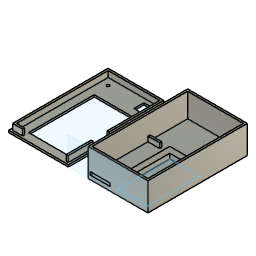
Untitled v1 (Autodesk Fusion 360 design; units mm, degrees)
Autodesk Fusion 360 part; units mm, degrees
sketch "Sketch1" plane through (0, 0, 0) normal (0, 0, 1) x (1, 0, 0)
  line L0 (0, 0) -> (76.2, 0)
  line L1 (76.2, 0) -> (76.2, 127)
  line L2 (76.2, 127) -> (0, 127)
  line L3 (0, 127) -> (0, 0)
  constraint horizontal L0
  constraint vertical L1
  constraint horizontal L2
  constraint vertical L3
  constraint coincident L0.start L3.end
extrude "Extrude1" add sketch "Sketch1" along normal blind 35.56 makes body 1
sketch "Sketch2" plane through (0, 0, 35.56) normal (0, 0, 1) x (-1, 0, 0)
  line L0 (0, -127) -> (0, 0)
  line L1 (0, 0) -> (-76.2, 0)
  line L2 (-76.2, 0) -> (-76.2, -127)
  line L3 (-76.2, -127) -> (0, -127)
  line L4 (-73.66, -124.46) -> (-2.54, -124.46)
  line L5 (-2.54, -124.46) -> (-2.54, -2.54)
  line L6 (-2.54, -2.54) -> (-73.66, -2.54)
  line L7 (-73.66, -2.54) -> (-73.66, -124.46)
  constraint horizontal L4
  constraint vertical L5
  constraint horizontal L6
  constraint vertical L7
extrude "Extrude2" cut sketch "Sketch2" against normal blind 30.48 contours L4 L5 L6 L7 bodies 1
sketch "Sketch3" plane through (0, 0, 0) normal (0, -1, 0) x (1, 0, 0)
  line L0 (0, 0) -> (76.2, 0)
  line L1 (76.2, 0) -> (76.2, 35.56)
  line L2 (76.2, 35.56) -> (0, 35.56)
  line L3 (0, 35.56) -> (0, 0)
sketch "Sketch4" plane through (0, 0, 0) normal (0, 0, 1) x (1, 0, 0)
move_body "Move1" bodies 1 to x (1, 0, 0) y (0, 1, 0) z (0, 0, 1) at (25.4, 0, 0)
sketch "Sketch5" plane through (0, 0, 0) normal (0, 0, 1) x (1, 0, 0)
  line L0 (0, 127) -> (-76.2, 127)
  line L1 (-76.2, 127) -> (-76.2, 0)
  line L2 (-76.2, 0) -> (0, 0)
  line L3 (0, 0) -> (0, 127)
  constraint horizontal L0
  constraint vertical L1
  constraint horizontal L2
  constraint vertical L3
extrude "Extrude3" add sketch "Sketch5" along normal blind 2.54 separate body makes body 2
sketch "Sketch6" plane through (0, 0, 2.54) normal (0, 0, 1) x (-1, 0, 0)
  line L0 (0, 0) -> (0, -127)
  line L1 (0, -127) -> (76.2, -127)
  line L2 (76.2, -127) -> (76.2, 0)
  line L3 (76.2, 0) -> (0, 0)
  line L4 (2.54, -2.54) -> (73.66, -2.54)
  line L5 (73.66, -2.54) -> (73.66, -124.46)
  line L6 (73.66, -124.46) -> (2.54, -124.46)
  line L7 (2.54, -124.46) -> (2.54, -2.54)
  constraint horizontal L4
  constraint vertical L5
  constraint horizontal L6
  constraint vertical L7
extrude "Extrude4" add sketch "Sketch6" along normal blind 7.62 contours L4 L5 L6 L7 bodies 2
sketch "Sketch7" plane through (0, 0, 10.16) normal (0, 0, 1) x (-1, 0, 0)
  line L0 (2.54, -124.46) -> (73.66, -124.46)
  line L1 (73.66, -124.46) -> (73.66, -2.54)
  line L2 (73.66, -2.54) -> (2.54, -2.54)
  line L3 (2.54, -2.54) -> (2.54, -124.46)
  line L4 (5.08, -5.08) -> (71.12, -5.08)
  line L5 (71.12, -5.08) -> (71.12, -121.92)
  line L6 (71.12, -121.92) -> (5.08, -121.92)
  line L7 (5.08, -121.92) -> (5.08, -5.08)
  constraint horizontal L4
  constraint vertical L5
  constraint horizontal L6
  constraint vertical L7
extrude "Extrude5" cut sketch "Sketch7" against normal blind 7.62 contours L4 L5 L6 L7 bodies 2
sketch "Sketch8" plane through (0, 0, 2.54) normal (0, 0, 1) x (-1, 0, 0)
  line L0 (5.08, -121.92) -> (71.12, -121.92)
  line L1 (71.12, -121.92) -> (71.12, -5.08)
  line L2 (71.12, -5.08) -> (5.08, -5.08)
  line L3 (5.08, -5.08) -> (5.08, -121.92)
sketch "Sketch9" plane through (0, 0, 10.16) normal (0, 0, 1) x (-1, 0, 0)
  line L0 (71.12, -5.08) -> (71.12, -121.92)
  line L1 (71.12, -121.92) -> (5.08, -121.92)
  line L2 (5.08, -121.92) -> (5.08, -5.08)
  line L3 (5.08, -5.08) -> (71.12, -5.08)
  line L4 (2.54, -124.46) -> (73.66, -124.46)
  line L5 (73.66, -124.46) -> (73.66, -2.54)
  line L6 (73.66, -2.54) -> (2.54, -2.54)
  line L7 (2.54, -2.54) -> (2.54, -124.46)
  line L8 (5.08, -2.54) -> (60.96, -2.54)
  line L9 (60.96, -2.54) -> (60.96, -5.08)
  line L10 (60.96, -5.08) -> (5.08, -5.08)
  line L11 (5.08, -5.08) -> (5.08, -2.54)
  constraint horizontal L8
  constraint vertical L9
  constraint horizontal L10
  constraint vertical L11
  constraint coincident L3 L9.end
  constraint coincident L6 L8.start
extrude "Extrude6" cut sketch "Sketch9" against normal blind 7.62 contours L3 L6 L8 L9 L10 L11 bodies 2
sketch "Sketch10" plane through (0, 0, 2.54) normal (0, 0, 1) x (-1, 0, 0)
  line L0 (2.54, -124.46) -> (2.54, -2.54)
  line L1 (2.54, -2.54) -> (5.08, -2.54)
  line L2 (5.08, -2.54) -> (5.08, -121.92)
  line L3 (5.08, -121.92) -> (71.12, -121.92)
  line L4 (71.12, -121.92) -> (71.12, -5.08)
  line L5 (71.12, -5.08) -> (60.96, -5.08)
  line L6 (60.96, -5.08) -> (60.96, -2.54)
  line L7 (60.96, -2.54) -> (73.66, -2.54)
  line L8 (73.66, -2.54) -> (73.66, -124.46)
  line L9 (73.66, -124.46) -> (2.54, -124.46)
  line L10 (0, 0) -> (0, -127)
  line L11 (0, -127) -> (76.2, -127)
  line L12 (76.2, -127) -> (76.2, 0)
  line L13 (76.2, 0) -> (0, 0)
  line L14 (5.08, -10.16) -> (60.96, -10.16)
  line L15 (60.96, -10.16) -> (60.96, -93.98)
  line L16 (60.96, -93.98) -> (5.08, -93.98)
  line L17 (5.08, -93.98) -> (5.08, -10.16)
  constraint horizontal L14
  constraint vertical L15
  constraint horizontal L16
  constraint vertical L17
  constraint coincident L2 L14.start
extrude "Extrude7" cut sketch "Sketch10" against normal blind 17.78 contours L2 L14 L15 L16 L17 bodies 2
sketch "Sketch11" plane through (0, 0, 0) normal (0, 0, -1) x (1, 0, 0)
  line L0 (-60.96, -93.98) -> (-60.96, -10.16)
  line L1 (-60.96, -10.16) -> (-5.08, -10.16)
  line L2 (-5.08, -10.16) -> (-5.08, -93.98)
  line L3 (-5.08, -93.98) -> (-60.96, -93.98)
  line L4 (0, -127) -> (0, 0)
  line L5 (0, 0) -> (-76.2, 0)
  line L6 (-76.2, 0) -> (-76.2, -127)
  line L7 (-76.2, -127) -> (0, -127)
  line L8 (-7.62, -116.84) -> (-20.32, -116.84)
  line L9 (-20.32, -116.84) -> (-20.32, -104.14)
  line L10 (-20.32, -104.14) -> (-7.62, -104.14)
  line L11 (-7.62, -104.14) -> (-7.62, -116.84)
  constraint horizontal L8
  constraint vertical L9
  constraint horizontal L10
  constraint vertical L11
extrude "Extrude8" cut sketch "Sketch11" against normal blind 7.62 contours L8 L9 L10 L11 bodies 2
sketch "Sketch12" plane through (0, 0, 0) normal (0, 0, -1) x (1, 0, 0)
  line L0 (-20.32, -116.84) -> (-20.32, -104.14)
  line L1 (-20.32, -104.14) -> (-7.62, -104.14)
  line L2 (-7.62, -104.14) -> (-7.62, -116.84)
  line L3 (-7.62, -116.84) -> (-20.32, -116.84)
  line L4 (-60.96, -93.98) -> (-60.96, -10.16)
  line L5 (-60.96, -10.16) -> (-5.08, -10.16)
  line L6 (-5.08, -10.16) -> (-5.08, -93.98)
  line L7 (-5.08, -93.98) -> (-60.96, -93.98)
  line L8 (0, -127) -> (0, 0)
  line L9 (0, 0) -> (-76.2, 0)
  line L10 (-76.2, 0) -> (-76.2, -127)
  line L11 (-76.2, -127) -> (0, -127)
  circle A0 centre (-62.23, -113.03) radius 1.778
extrude "Extrude9" cut sketch "Sketch12" against normal blind 7.62 contours A0 bodies 2
sketch "Sketch13" plane through (0, 0, 5.08) normal (0, 0, 1) x (-1, 0, 0)
  line L0 (-99.06, -2.54) -> (-99.06, -124.46)
  line L1 (-99.06, -124.46) -> (-27.94, -124.46)
  line L2 (-27.94, -124.46) -> (-27.94, -2.54)
  line L3 (-27.94, -2.54) -> (-99.06, -2.54)
sketch "Sketch14" plane through (0, 0, 0) normal (0, -1, 0) x (1, 0, 0)
  line L0 (25.4, 0) -> (101.6, 0)
  line L1 (101.6, 0) -> (101.6, 35.56)
  line L2 (101.6, 35.56) -> (25.4, 35.56)
  line L3 (25.4, 35.56) -> (25.4, 0)
sketch "Sketch15" plane through (0, 2.54, 0) normal (0, 1, 0) x (-1, 0, 0)
  line L0 (-27.94, 35.56) -> (-99.06, 35.56)
  line L1 (-99.06, 35.56) -> (-99.06, 5.08)
  line L2 (-99.06, 5.08) -> (-27.94, 5.08)
  line L3 (-27.94, 5.08) -> (-27.94, 35.56)
  line L4 (-27.94, 5.08) -> (-53.34, 5.08)
  line L5 (-53.34, 5.08) -> (-53.34, 8.89)
  line L6 (-53.34, 8.89) -> (-27.94, 8.89)
  line L7 (-27.94, 8.89) -> (-27.94, 5.08)
  constraint horizontal L4
  constraint vertical L5
  constraint horizontal L6
  constraint vertical L7
  constraint coincident L2.end L3.start
extrude "Extrude10" cut sketch "Sketch15" against normal blind 13.97 contours L2 L3 L4 L5 L6 L7 bodies 1
sketch "Sketch16" plane through (0, 0, 5.08) normal (0, 0, 1) x (-1, 0, 0)
  line L0 (-53.34, -2.54) -> (-55.88, -2.54)
  line L1 (-55.88, -2.54) -> (-55.88, -73.66)
  line L2 (-55.88, -73.66) -> (-53.34, -73.66)
  line L3 (-53.34, -73.66) -> (-53.34, -2.54)
  constraint horizontal L0
  constraint vertical L1
  constraint horizontal L2
  constraint vertical L3
extrude "Extrude11" add sketch "Sketch16" along normal blind 6.35 bodies 1
sketch "Sketch17" plane through (0, 0, 5.08) normal (0, 0, 1) x (-1, 0, 0)
  line L0 (-55.88, -73.66) -> (-27.94, -73.66)
  line L1 (-27.94, -73.66) -> (-27.94, -76.2)
  line L2 (-27.94, -76.2) -> (-55.88, -76.2)
  line L3 (-55.88, -76.2) -> (-55.88, -73.66)
  constraint horizontal L0
  constraint vertical L1
  constraint horizontal L2
  constraint vertical L3
extrude "Extrude12" add sketch "Sketch17" along normal blind 6.35 bodies 1
sketch "Sketch18" plane through (0, 0, 11.43) normal (0, 0, 1) x (-1, 0, 0)
  line L0 (-53.34, -73.66) -> (-53.34, -2.54)
  line L1 (-53.34, -2.54) -> (-55.88, -2.54)
  line L2 (-55.88, -2.54) -> (-55.88, -76.2)
  line L3 (-55.88, -76.2) -> (-27.94, -76.2)
  line L4 (-27.94, -76.2) -> (-27.94, -73.66)
  line L5 (-27.94, -73.66) -> (-53.34, -73.66)
  line L6 (-53.34, -73.66) -> (-43.18, -73.66)
  line L7 (-43.18, -73.66) -> (-43.18, -76.2)
  line L8 (-43.18, -76.2) -> (-53.34, -76.2)
  line L9 (-53.34, -76.2) -> (-53.34, -73.66)
  constraint horizontal L6
  constraint vertical L7
  constraint horizontal L8
  constraint vertical L9
  constraint coincident L3 L7.end
  constraint coincident L0.start L5.end
extrude "Extrude13" cut sketch "Sketch18" against normal blind 6.35 contours L3 L5 L6 L7 L8 L9 bodies 1
sketch "Sketch19" plane through (0, 0, 5.08) normal (0, 0, 1) x (-1, 0, 0)
  line L0 (-99.06, -2.54) -> (-60.96, -2.54)
  line L1 (-60.96, -2.54) -> (-60.96, -68.58)
  line L2 (-60.96, -68.58) -> (-99.06, -68.58)
  line L3 (-99.06, -68.58) -> (-99.06, -2.54)
  constraint horizontal L0
  constraint vertical L1
  constraint horizontal L2
  constraint vertical L3
extrude "Extrude14" add 1 faces at (55.88, 27.0933, 9.3133) along direction (1, 0, 0) blind 5.08 on bodies 1 bodies 1
sketch "Sketch20" plane through (60.96, 0, 0) normal (1, 0, 0) x (0, 1, 0)
  line L0 (2.54, 5.08) -> (76.2, 5.08)
  line L1 (76.2, 5.08) -> (76.2, 11.43)
  line L2 (76.2, 11.43) -> (2.54, 11.43)
  line L3 (2.54, 11.43) -> (2.54, 5.08)
  line L4 (76.2, 11.43) -> (68.58, 11.43)
  line L5 (68.58, 11.43) -> (68.58, 5.08)
  line L6 (68.58, 5.08) -> (76.2, 5.08)
  line L7 (76.2, 5.08) -> (76.2, 11.43)
  constraint horizontal L4
  constraint vertical L5
  constraint horizontal L6
  constraint vertical L7
  constraint coincident L0 L5.end
  constraint coincident L1.end L2.start
extrude "Extrude15" add sketch "Sketch20" along normal blind 38.1 contours L0 L1 L2 L4 L5 L6 L7 bodies 1
sketch "Sketch21" plane through (-5.08, 0, 0) normal (-1, 0, 0) x (0, -1, 0)
  line L0 (-2.54, 10.16) -> (-121.92, 10.16)
  line L1 (-121.92, 10.16) -> (-121.92, 2.54)
  line L2 (-121.92, 2.54) -> (-93.98, 2.54)
  line L3 (-93.98, 2.54) -> (-93.98, 0)
  line L4 (-93.98, 0) -> (-10.16, 0)
  line L5 (-10.16, 0) -> (-10.16, 2.54)
  line L6 (-10.16, 2.54) -> (-2.54, 2.54)
  line L7 (-2.54, 2.54) -> (-2.54, 10.16)
  line L8 (-34.29, 2.54) -> (-34.29, 10.16)
  line L9 (-34.29, 10.16) -> (-10.16, 10.16)
  line L10 (-34.29, 2.54) -> (-54.61, 2.54)
  line L11 (-54.61, 2.54) -> (-54.61, 10.16)
  line L12 (-54.61, 10.16) -> (-34.29, 10.16)
  line L13 (-34.29, 10.16) -> (-34.29, 2.54)
  constraint vertical L8
  constraint horizontal L9
  constraint coincident L0 L8.end
  constraint horizontal L10
  constraint vertical L11
  constraint horizontal L12
  constraint vertical L13
  constraint coincident L0 L11.end
extrude "Extrude16" cut sketch "Sketch21" against normal blind 2.54 contours L0 L8 L10 L11 L12 L13 bodies 2
